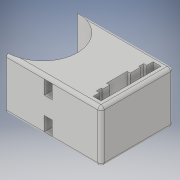
# Autodesk Inventor part: rear_light_mount
Saved by Autodesk Inventor 2019 (Build 230136000, 136)
## iProperties
Created: 2019-09-25
Part Number: rear_light_mount
Material: Generic
Document SubType Name: Modeling
Designer: Alex
Density: 1 g/cm^3
Appearance: Default
Author: Alex
Autodesk Inventor part; units mm, degrees
ref_plane "YZ Plane" through (0, 0, 0) normal (1, 0, 0) x (0, 1, 0)
ref_plane "XZ Plane" through (0, 0, 0) normal (0, 1, 0) x (-1, 0, 0)
ref_plane "XY Plane" through (0, 0, 0) normal (0, 0, 1) x (1, 0, 0)
sketch "Sketch1" plane through (0, 0, 0) normal (0, 1, 0) x (-1, 0, 0)
  line L0 (162, 9) -> (164.5, 9)
  line L1 (164.5, -10) -> (162, -10)
  line L2 (162, -10) -> (162, 9)
  line L3 (190, 11) -> (161, 11)
  line L4 (160, 10) -> (160, -11)
  line L5 (161, -12) -> (190, -12)
  line L6 (164.5, 7) -> (165.5, 7)
  line L7 (164.5, -8) -> (165.5, -8)
  line L8 (165.5, 7) -> (165.5, 5.5)
  line L9 (165.5, 5.5) -> (165, 5.5)
  line L10 (165.5, -8) -> (165.5, -6.5)
  line L11 (165.5, -6.5) -> (165, -6.5)
  line L12 (164.5, 7) -> (164.5, 9)
  line L13 (165, 5.5) -> (165, -6.5)
  line L14 (164.5, -8) -> (164.5, -10)
  arc A0 (161, 11) -> (160, 10) centre (161, 10) ccw
  arc A1 (160, -11) -> (161, -12) centre (161, -11) ccw
  line L15 (190, 11) -> (190, -12)
  point P0 (0, 0)
  dimension "d0" = 19
  dimension "d1" = 2.5
  dimension "d3" = 2
  dimension "d4" = 2
  dimension "d5" = 2
  dimension "d7" = 1
  dimension "d8" = 15
  dimension "d10" = 1.5
  dimension "d11" = 1.5
  dimension "d12" = 1
  dimension "d22" = 4
  dimension "d28" = 3
  dimension "d36" = 30
  dimension "d46" = 11
  dimension "d48" = 190
  constraints: 32 end point, 4 parallel, 4 point on circle, 4 tangent, 3 horizontal, 3 vertical, 2 centre point, 1 equal radius, 1 perpendicular, 1 point on line
  measures "d0" distance of L0.end L1.start
  measures "d1" distance of L1.start L1.end
  measures "d3" distance between parallel lines of L4 L2
  measures "d4" distance between parallel lines of L3 L0
  measures "d5" distance between parallel lines of L5 L1
  measures "d7" distance of L6.start L6.end
  measures "d8" distance between parallel lines of L7 L6
  measures "d10" distance of L6.end L8.end
  measures "d11" distance of L7.end L10.end
  measures "d12" radius of A0
  measures "d22" distance between parallel lines of L5 L7
  measures "d28" distance between parallel lines of L2 L13
  measures "d36" distance between parallel lines of L15 L4
  measures "d46" distance from line of point (0, 0) L3
  measures "d48" distance from line of point (0, 0) L15
extrude "Extrusion1" add sketch "Sketch1" along normal blind 16.5
sketch "Sketch5" plane through (0, 16.5, 0) normal (0, 1, 0) x (1, 0, 0)
  line L0 (-165, -3.25) -> (-166, -3.25)
  line L1 (-166, -3.25) -> (-166, 3.25)
  line L2 (-166, 3.25) -> (-165, 3.25)
  line L3 (-165, 3.25) -> (-165, -3.25)
  line L4 (-165, -5.5) -> (-165, 6.5) projected
  line L5 (-190, -11) -> (-161, -11) projected
  point P0 (0, 0)
  point P1 (-21.5, -2)
  dimension "d15" = 1
  dimension "d16" = 6.5
  dimension "d17" = 0
  dimension "d18" = 7.75
  constraints: 8 end point, 2 parallel, 1 horizontal, 1 perpendicular, 1 other
  measures "d15" distance between parallel lines of L1 L3
  measures "d16" distance between parallel lines of L2 L0
  measures "d17" distance between parallel lines of L4 L3
extrude "Extrusion2" cut sketch "Sketch5" against normal blind 15
move or copy body "Move Body2" bodies to move or copy 1 copy no translate (63, 210, 0)
fillet "Fillet1" [suppressed]
sketch "Sketch21" plane through (-127, 226.5, 11) normal (0, 1, 0) x (1, 0, 0)
  circle A0 centre (0, 11.5) radius 11
  line L0 (24, 7.75) -> (24, 14.25) projected
  line L1 (29, 23) -> (0, 23) projected
  circle A1 centre (0, 11.5) radius 13
  line L2 (0, 0) -> (29, 0) projected
  point P0 (127, 11)
  point P1 (6.0622, 0)
  dimension "d61" = 26
  dimension "d56" = 22
  dimension "d57" = 24
  dimension "d58" = 11.5
  constraints: 1 centre point, 1 coincident, 1 point on line, 3 other
  measures "d56" diameter of A0
  measures "d57" distance from line of L0 A0.centre
  measures "d58" distance from line of L1 A0.centre
extrude "Extrusion4" cut sketch "Sketch21" against normal up to next contours A0
sketch "Sketch24" plane through (-98, 210, -12) normal (0, 0, -1) x (-1, 0, 0)
  line L0 (17, 1) -> (14.5, 1)
  line L1 (14.5, 1) -> (14.5, 5.5)
  line L2 (14.5, 5.5) -> (17, 5.5)
  line L3 (17, 5.5) -> (17, 1)
  line L4 (17, 11.1) -> (14.5, 11.1)
  line L5 (14.5, 11.1) -> (14.5, 15.5)
  line L6 (14.5, 15.5) -> (17, 15.5)
  line L7 (17, 15.5) -> (17, 11.1)
  line L8 (29, 0) -> (0, 0) projected
  line L9 (29, 0) -> (29, 16.5) projected
  line L10 (0, 16.5) -> (29, 16.5) projected
  point P0 (-98, -210)
  dimension "d68" = 2.5
  dimension "d69" = 4.5
  dimension "d70" = 2.5
  dimension "d71" = 4.4
  dimension "d72" = 1
  dimension "d73" = 12
  dimension "d74" = 12
  dimension "d75" = 1
  constraints: 16 end point, 4 parallel, 2 horizontal, 2 perpendicular
  measures "d68" distance of L1.end L2.end
  measures "d69" distance of L0.end L1.end
  measures "d70" distance of L5.end L6.end
  measures "d71" distance of L4.end L5.end
  measures "d72" distance between parallel lines of L8 L0
  measures "d73" distance between parallel lines of L9 L3
  measures "d74" distance between parallel lines of L9 L7
  measures "d75" distance between parallel lines of L10 L6
extrude "Extrusion5" cut sketch "Sketch24" against normal up to next
fillet "Fillet2" radius 1 10 edges at (-97.2929, 210, -11.7071) (-97, 210, -0.5) (-97.2929, 210, 10.7071) (-112.5, 210, 11) (-112.5, 210, -12) (-97.2929, 226.5, -11.7071) (-97, 226.5, -0.5) (-97.2929, 226.5, 10.7071) (-112.5, 226.5, 11) (-112.5, 226.5, -12)
body "Solid1"
